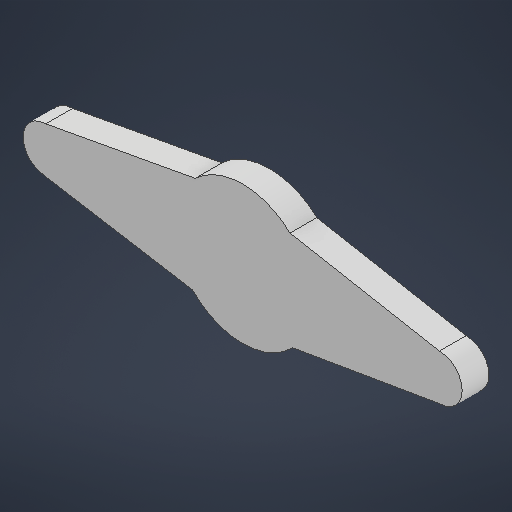
# Autodesk Inventor part: servo_motor_header
Saved by Autodesk Inventor 2026 (Build 300175000, 175)
## iProperties
Created: 2025-06-29
Part Number: servo_motor_header
Material: Generic
Document SubType Name: Modeling
Designer: user
Density: 1 g/cm^3
Appearance: Default
Author: user
Autodesk Inventor part; units mm, degrees
ref_plane "YZ Plane" through (0, 0, 0) normal (1, 0, 0) x (0, 1, 0)
ref_plane "XZ Plane" through (0, 0, 0) normal (0, 1, 0) x (-1, 0, 0)
ref_plane "XY Plane" through (0, 0, 0) normal (0, 0, 1) x (1, 0, 0)
sketch "Sketch1" plane through (0, 0, 0) normal (0, 0, 1) x (1, 0, 0)
  circle A0 centre (-80.5407, 0) radius 2.125
  circle A1 centre (-43.7907, 0) radius 2.125
  circle A2 centre (-62.1657, 0) radius 6.45
  line L0 (-62.1657, 0) -> (-43.7907, 0)
  line L1 (-80.5407, 0) -> (-62.1657, 0)
  line L2 (-80.5407, 2.125) -> (-66.5913, 4.6922)
  line L3 (-80.8923, -2.0957) -> (-66.8303, -4.4547)
  line L4 (-43.7907, 2.125) -> (-57.7402, 4.6922)
  line L5 (-43.7907, -2.125) -> (-57.5041, -4.4578)
  point P0 (0, 0)
  dimension "d0" = 4.25
  dimension "d1" = 4.25
  dimension "d2" = 41
  dimension "d3" = 12.9
  dimension "d4" = 9.15
  dimension "d5" = 9.15
  constraints: 12 end point, 8 point on circle, 3 centre point, 2 horizontal, 1 collinear, 1 tangent
  measures "d0" diameter of A0
  measures "d1" diameter of A1
  measures "d3" diameter of A2
  measures "d4" distance of L3.end L2.end
  measures "d5" vertical distance of L5.end L4.end
extrude "Extrusion1" add sketch "Sketch1" along normal blind 2.5
sketch "Sketch2" plane through (0, 0, 0) normal (0, 0, -1) x (-1, 0, 0)
  arc A0 (66.5913, 4.6922) -> (57.7402, 4.6922) centre (62.1657, 0) ccw projected
  circle A1 centre (62.1657, 0) radius 2.75
  point P0 (0, 0)
  dimension "d8" = 5.5
  constraints: 1 centre point, 1 coincident
  measures "d8" diameter of A1
extrude "Extrusion2" cut sketch "Sketch2" against normal blind 2.3
body "Solid1"
